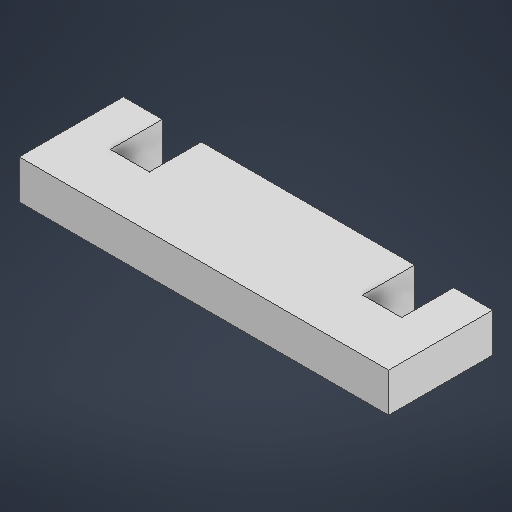
# Autodesk Inventor part: upper support
Saved by Autodesk Inventor 2025.3 (Build 293356030, 356C)
## iProperties
Created: 2025-09-05
Part Number: upper support
Material: 一般
Document SubType Name: Modeling
Designer: 陳泓任
Density: 1 g/cm^3
Appearance: 預設
Author: 陳泓任
Autodesk Inventor part; units mm, degrees
ref_plane "YZ Plane" through (0, 0, 0) normal (1, 0, 0) x (0, 1, 0)
ref_plane "XZ Plane" through (0, 0, 0) normal (0, 1, 0) x (-1, 0, 0)
ref_plane "XY Plane" through (0, 0, 0) normal (0, 0, 1) x (1, 0, 0)
sketch "草圖1" plane through (0, 0, 0) normal (0, 1, 0) x (-1, 0, 0)
  line L0 (-14.2, 4) -> (14.2, 4)
  line L1 (14.2, 4) -> (14.2, -4)
  line L2 (-14.2, -4) -> (-14.2, 4)
  line L3 (-14.2, 4) -> (14.2, -4) construction
  line L4 (14.2, 4) -> (-14.2, -4) construction
  line L5 (-11.2, -4) -> (-11.2, 0)
  line L6 (-11.2, 0) -> (-8.2, 0)
  line L7 (-8.2, 0) -> (-8.2, -4)
  line L8 (0, 7.3969) -> (0, -7.2649)
  line L9 (11.2, -4) -> (11.2, 0)
  line L10 (11.2, 0) -> (8.2, 0)
  line L11 (8.2, 0) -> (8.2, -4)
  line L12 (14.2, -4) -> (11.2, -4)
  line L13 (8.2, -4) -> (-8.2, -4)
  line L14 (-11.2, -4) -> (-14.2, -4)
  point P0 (0, 0)
  dimension "d0" = 4
  dimension "d1" = 8
  dimension "d2" = 16.4
  dimension "d3" = 3
  dimension "d5" = 28.4
  constraints: 30 end point, 5 perpendicular, 4 parallel, 4 symmetric about line, 2 midpoint, 2 vertical, 1 collinear, 1 horizontal, 1 point on line
  measures "d0" distance of L5.start L5.end
  measures "d1" distance of L2.start L0.start
  measures "d2" diameter of L7 L8
  measures "d3" distance of L5.end L6.end
  measures "d5" diameter of L2 L8
extrude "擠出1" add sketch "草圖1" along normal blind 3
equation "\"d5\" = d2 + 4 * d3"
